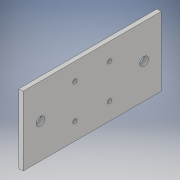
# Autodesk Inventor part: 2AM-17-P-0206  - slider plate
Saved by Autodesk Inventor 2017 (Build 210142000, 142)
## iProperties
Created: 2017-12-27
Part Number: 2AM-17-P-0206  - slider plate
Material: Generic
Document SubType Name: Modeling
Designer: Micah
Density: 1 g/cm^3
Appearance: Default
Author: Micah
Autodesk Inventor part; units mm, degrees
ref_plane "YZ Plane" through (0, 0, 0) normal (1, 0, 0) x (0, 1, 0)
ref_plane "XZ Plane" through (0, 0, 0) normal (0, 1, 0) x (-1, 0, 0)
ref_plane "XY Plane" through (0, 0, 0) normal (0, 0, 1) x (1, 0, 0)
sketch "Sketch1" plane through (0, 0, 0) normal (1, 0, 0) x (0, 1, 0)
  line L0 (0, 0) -> (50.8, 0)
  line L1 (50.8, 0) -> (50.8, 101.6)
  line L2 (50.8, 101.6) -> (0, 101.6)
  line L3 (0, 101.6) -> (0, 0)
  line L4 (50.8, 0) -> (50.8, 12.7) construction
  line L5 (50.8, 12.7) -> (0, 12.7) construction
  line L6 (25.4, 0) -> (25.4, 12.7) construction
  circle A0 centre (25.4, 12.7) radius 3.175
  line L7 (50.8, 12.7) -> (50.8, 38.1) construction
  line L8 (50.8, 38.1) -> (38.1, 38.1) construction
  circle A1 centre (38.1, 38.1) radius 1.5875
  line L9 (0, 38.1) -> (12.7, 38.1) construction
  circle A2 centre (12.7, 38.1) radius 1.5875
  line L10 (50.8, 50.8) -> (0, 50.8) construction
  circle A3 centre (25.4, 88.9) radius 3.175
  circle A4 centre (38.1, 63.5) radius 1.5875
  circle A5 centre (12.7, 63.5) radius 1.5875
  dimension "d11" = 50.8
  dimension "d12" = 101.6
  dimension "d13" = 12.7
  dimension "d14" = 6.35
  dimension "d15" = 25.4
  dimension "d16" = 12.7
  dimension "d17" = 3.175
  dimension "d18" = 12.7
  dimension "d19" = 3.175
  constraints: 22 end point, 6 centre point, 4 midpoint, 4 point on line, 3 coincident, 3 perpendicular, 3 symmetric about line, 2 horizontal, 2 parallel, 3 other
  measures "d11" distance of L2.end L1.end
  measures "d12" distance of L1.end L0.end
  measures "d13" distance of L0.end L4.end
  measures "d14" diameter of A0
  measures "d15" distance of L4.end L7.end
  measures "d16" distance of L7.end L8.end
  measures "d17" diameter of A1
  measures "d18" distance of L9.start L9.end
  measures "d19" diameter of A2
extrude "Extrusion1" add sketch "Sketch1" along normal blind 3.175
body "Solid1"
